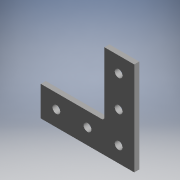
# Autodesk Inventor part: 25-4081 Aluminum
Saved by Autodesk Inventor 2019.4 (Build 234330000, 330)
## iProperties
Category: PARTsolutions
Company: 8020
Part Number: 25-4081 Aluminum
Material: Generic
Catalog Web Link: www.cadenas.de
Description: 20-4081, 25-4081, 30-4481, 40-4481, 45-4481, 20-4081-Black, 25-4081-Black, 30-4481-Black, 40-4481-Black, 45-4481-Black-5 Hole - "L" Flat Plate
Vendor: 8020
Document SubType Name: Modeling
Designer: partserver
Manufacturer: 8020
Mass: 11.476 g
Surface Area: 73.304 cm^2
Volume: 11.476 cm^3
Density: 1 g/cm^3
Appearance: PSOLRGB-191-191-191
PSOL_IDENT_0: {$CADENAS_DATA\23d-libs\8020\metric\joining_plates\20_4081.prj},266 {VTYP=3D},{NB=25-4081},{LINA=25-
PSOL_IDENT_1: 4081},{NN=20-4081, 25-4081, 30-4481, 40-4481, 45-4481, 20-4081-Black, 25-4081-Black, 30-4481-Black,
PSOL_IDENT_2: 40-4481-Black, 45-4481-Black},{DATE=31.07.2020 09:21:28},{GEOMDATE=22.01.2019 19:48:00},{VERSION=},{
PSOL_IDENT_3: LINEID=60},{WBVAR=},{WBNUMERIC=}  {NB=25-4081},{LINA=25-4081},{KT=DUMMY},{PN=25-4081},{SERIES=25},{M
PSOL_IDENT_4: ATERIAL=Aluminum},{GRADE=6105-T5},{FINISH=Clear Anodize},{A=75.0},{B=75.0},{C=25.0},{D=12.5},{E=6.30
PSOL_IDENT_5: },{F=4.0},{G=24.0},{H=24.0},{J=2.0},{WEIGHT=.030},{COLOR=.75,.75,.75}
NB: 25-4081
NN: 20-4081, 25-4081, 30-4481, 40-4481, 45-4481, 20-4081-Black, 25-4081-Black, 30-4481-Black, 40-4481-Black, 45-4481-Black
NT: 5 Hole - "L" Flat Plate
NBSYN: $PN.
LINA: 25-4081
CATALOG: 80/20
PN: 25-4081
SERIES: 25
MATERIAL: Aluminum
GRADE: 6105-T5
FINISH: Clear Anodize
A: 75
B: 75
C: 25
D: 12.5
E: 6.3
F: 4
G: 24
H: 24
J: 2
WEIGHT: .030
SUPPLIER: 8020
ARTICLENO: 25-4081
BOMINFO: 25-4081
CREATOR: CADENAS GmbH
Title: 25-4081
Author: Cadenas PARTsolutions
Comments: 5 Hole - "L" Flat Plate
Autodesk Inventor part; units mm, degrees
ref_plane "YZ Plane" through (0, 0, 0) normal (1, 0, 0) x (0, 1, 0)
ref_plane "XZ Plane" through (0, 0, 0) normal (0, 1, 0) x (-1, 0, 0)
ref_plane "XY Plane" through (0, 0, 0) normal (0, 0, 1) x (1, 0, 0)
sketch "Sketch_1" plane through (0, 0, 0) normal (0, 1, 0) x (-1, 0, 0)
  line L0 (0, 0) -> (-75, 0)
  line L1 (-75, 0) -> (-75, -24)
  line L2 (-75, -24) -> (-26, -24)
  arc A0 (-24, -26) -> (-26, -24) centre (-26, -26) ccw
  line L3 (-24, -26) -> (-24, -75)
  line L4 (-24, -75) -> (0, -75)
  line L5 (0, -75) -> (0, 0)
  circle A1 centre (-62.5, -12.5) radius 3.15
  circle A2 centre (-37.5, -12.5) radius 3.15
  circle A3 centre (-12.5, -12.5) radius 3.15
  circle A4 centre (-12.5, -37.5) radius 3.15
  circle A5 centre (-12.5, -62.5) radius 3.15
  constraints: 12 end point, 6 centre point, 2 point on circle
extrude "Extrusion1" add sketch "Sketch_1" along normal blind 4
body "Solid1"
